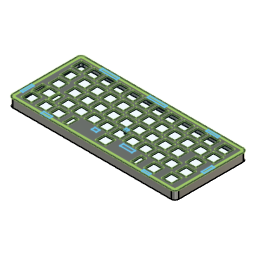
RowLow52V2-topcase v4 (Autodesk Fusion 360 design; units mm, degrees)
Autodesk Fusion 360 part; units mm, degrees
sketch "スケッチ1" plane through (0, 0, 0) normal (0, 0, 1) x (1, 0, 0)
  spline S0 degree 3 poles (2.4631, -100.8553) (0.8767, -100.8553) (-0.441, -99.5645) (-0.4745, -97.9777) knots 0 0 0 0 1 1 1 1
  line L0 (-0.4745, -97.9777) -> (-0.4745, -2.5093)
  spline S1 degree 3 poles (-0.4745, -2.5093) (-0.5048, -0.9017) (0.7856, 0.4413) (2.4031, 0.4748) knots 0 0 0 0 1 1 1 1
  line L1 (2.4031, 0.4748) -> (236.6144, 0.4695)
  spline S2 degree 3 poles (236.6144, 0.4695) (238.2009, 0.4695) (239.5181, -0.8213) (239.5513, -2.4081) knots 0 0 0 0 1 1 1 1
  line L2 (239.5513, -2.4081) -> (239.5337, -97.857)
  spline S3 degree 3 poles (239.5337, -97.857) (239.5643, -99.4643) (238.2739, -100.807) (236.6571, -100.8412) knots 0 0 0 0 1 1 1 1
  line L3 (236.6571, -100.8412) -> (2.4631, -100.8553)
  spline S4 degree 3 poles (2.4631, -103.3551) (-0.4734, -103.3554) (-2.9122, -100.9664) (-2.9739, -98.0302) knots 0 0 0 0 1 1 1 1
  line L4 (-2.9739, -98.0302) -> (-2.9746, -2.534)
  spline S5 degree 3 poles (-2.9746, -2.534) (-3.0134, 0.4445) (-0.6311, 2.9125) (2.3509, 2.9743) knots 0 0 0 0 1 1 1 1
  line L5 (2.3509, 2.9743) -> (236.614, 2.9697)
  spline S6 degree 3 poles (236.614, 2.9697) (239.5506, 2.9697) (241.9893, 0.5807) (242.0503, -2.3562) knots 0 0 0 0 1 1 1 1
  line L6 (242.0503, -2.3562) -> (242.0334, -97.8351)
  spline S7 degree 3 poles (242.0334, -97.8351) (242.0712, -100.8119) (239.6896, -103.2781) (236.7089, -103.3406) knots 0 0 0 0 1 1 1 1
  line L7 (236.7089, -103.3406) -> (2.4631, -103.3551)
  line L8 (239.0514, -2.4183) -> (239.0338, -97.857)
  spline S8 degree 3 poles (239.0338, -97.857) (239.0592, -99.2018) (237.9909, -100.3131) (236.6461, -100.3413) knots 0 0 0 0 1 1 1 1
  line L9 (236.6461, -100.3413) -> (2.51, -100.3547)
  spline S9 degree 3 poles (2.51, -100.3547) (1.1649, -100.3801) (0.0536, -99.3119) (0.0254, -97.9671) knots 0 0 0 0 1 1 1 1
  line L10 (0.0254, -97.9671) -> (0.0254, -2.5093)
  spline S10 degree 3 poles (0.0254, -2.5093) (0, -1.1645) (1.0682, -0.0529) (2.4134, -0.025) knots 0 0 0 0 1 1 1 1
  line L11 (2.4134, -0.025) -> (236.5671, -0.031)
  spline S11 degree 3 poles (236.5671, -0.031) (237.9119, -0.0053) (239.0235, -1.0739) (239.0514, -2.4183) knots 0 0 0 0 1 1 1 1
  line L12 (131.3131, -95.1177) -> (117.2132, -95.1177)
  line L13 (117.2132, -95.1177) -> (117.2132, -81.0175)
  line L14 (117.2132, -81.0175) -> (131.3131, -81.0175)
  line L15 (131.3131, -81.0175) -> (131.3131, -95.1177)
  line L16 (177.7735, -96.8678) -> (170.7734, -96.8678)
  line L17 (170.7734, -96.8678) -> (170.7734, -82.0678)
  line L18 (170.7734, -82.0678) -> (177.7735, -82.0678)
  line L19 (177.7735, -82.0678) -> (177.7735, -96.8678)
  line L20 (70.7531, -96.8678) -> (77.7533, -96.8678)
  line L21 (77.7533, -96.8678) -> (77.7533, -82.0678)
  line L22 (77.7533, -82.0678) -> (70.7531, -82.0678)
  line L23 (70.7531, -82.0678) -> (70.7531, -96.8678)
  line L24 (28.9193, -76.0677) -> (14.8195, -76.0677)
  line L25 (14.8195, -76.0677) -> (14.8195, -61.9675)
  line L26 (14.8195, -61.9675) -> (28.9197, -61.9675)
  line L27 (28.9197, -61.9675) -> (28.9193, -76.0677)
  line L28 (37.2696, -77.8178) -> (30.2694, -77.8178)
  line L29 (30.2694, -77.8178) -> (30.2694, -63.0178)
  line L30 (30.2694, -63.0178) -> (37.2696, -63.0178)
  line L31 (37.2696, -63.0178) -> (37.2696, -77.8178)
  line L32 (6.4696, -77.8178) -> (13.4698, -77.8178)
  line L33 (13.4698, -77.8178) -> (13.4698, -63.0178)
  line L34 (13.4698, -63.0178) -> (6.4696, -63.0178)
  line L35 (6.4696, -63.0178) -> (6.4696, -77.8178)
  line L36 (226.5634, -57.0177) -> (212.4632, -57.0177)
  line L37 (212.4632, -57.0177) -> (212.4632, -42.9175)
  line L38 (212.4632, -42.9175) -> (226.5634, -42.9175)
  line L39 (226.5634, -42.9175) -> (226.5634, -57.0177)
  line L40 (228.9443, -95.1177) -> (214.8445, -95.1177)
  line L41 (214.8445, -95.1177) -> (214.8445, -81.0175)
  line L42 (214.8445, -81.0175) -> (228.9443, -81.0175)
  line L43 (228.9443, -81.0175) -> (228.9443, -95.1177)
  line L44 (24.1568, -57.0177) -> (10.057, -57.0177)
  line L45 (10.057, -57.0177) -> (10.057, -42.9175)
  line L46 (10.057, -42.9175) -> (24.1572, -42.9175)
  line L47 (24.1572, -42.9175) -> (24.1568, -57.0177)
  line L48 (21.7756, -37.9677) -> (7.6761, -37.9677)
  line L49 (7.6761, -37.9677) -> (7.6761, -23.8675)
  line L50 (7.6761, -23.8675) -> (21.7759, -23.8675)
  line L51 (21.7759, -23.8675) -> (21.7756, -37.9677)
  line L52 (21.7756, -95.1177) -> (7.6761, -95.1177)
  line L53 (7.6761, -95.1177) -> (7.6761, -81.0175)
  line L54 (7.6761, -81.0175) -> (21.7759, -81.0175)
  line L55 (21.7759, -81.0175) -> (21.7756, -95.1177)
  line L56 (231.3259, -18.9177) -> (217.2257, -18.9177)
  line L57 (217.2257, -18.9177) -> (217.2257, -4.8175)
  line L58 (217.2257, -4.8175) -> (231.3259, -4.8175)
  line L59 (231.3259, -4.8175) -> (231.3259, -18.9177)
  line L60 (202.7509, -95.1177) -> (188.6507, -95.1177)
  line L61 (188.6507, -95.1177) -> (188.6507, -81.0175)
  line L62 (188.6507, -81.0175) -> (202.7509, -81.0175)
  line L63 (202.7509, -81.0175) -> (202.7509, -95.1177)
  line L64 (231.3259, -76.0677) -> (217.2257, -76.0677)
  line L65 (217.2257, -76.0677) -> (217.2257, -61.9675)
  line L66 (217.2257, -61.9675) -> (231.3259, -61.9675)
  line L67 (231.3259, -61.9675) -> (231.3259, -76.0677)
  line L68 (214.6568, -37.9677) -> (200.557, -37.9677)
  line L69 (200.557, -37.9677) -> (200.557, -23.8675)
  line L70 (200.557, -23.8675) -> (214.6568, -23.8675)
  line L71 (214.6568, -23.8675) -> (214.6568, -37.9677)
  line L72 (57.4943, -18.9177) -> (43.3941, -18.9177)
  line L73 (43.3941, -18.9177) -> (43.3941, -4.8175)
  line L74 (43.3941, -4.8175) -> (57.4943, -4.8175)
  line L75 (57.4943, -4.8175) -> (57.4943, -18.9177)
  line L76 (152.7443, -18.9177) -> (138.6441, -18.9177)
  line L77 (138.6441, -18.9177) -> (138.6441, -4.8175)
  line L78 (138.6441, -4.8175) -> (152.7443, -4.8175)
  line L79 (152.7443, -4.8175) -> (152.7443, -18.9177)
  line L80 (95.5943, -76.0677) -> (81.4941, -76.0677)
  line L81 (81.4941, -76.0677) -> (81.4941, -61.9675)
  line L82 (81.4941, -61.9675) -> (95.5943, -61.9675)
  line L83 (95.5943, -61.9675) -> (95.5943, -76.0677)
  line L84 (162.2693, -57.0177) -> (148.1691, -57.0177)
  line L85 (148.1691, -57.0177) -> (148.1691, -42.9175)
  line L86 (148.1691, -42.9175) -> (162.2693, -42.9175)
  line L87 (162.2693, -42.9175) -> (162.2693, -57.0177)
  line L88 (114.6443, -18.9177) -> (100.5441, -18.9177)
  line L89 (100.5441, -18.9177) -> (100.5441, -4.8175)
  line L90 (100.5441, -4.8175) -> (114.6443, -4.8175)
  line L91 (114.6443, -4.8175) -> (114.6443, -18.9177)
  line L92 (138.4568, -37.9677) -> (124.3566, -37.9677)
  line L93 (124.3566, -37.9677) -> (124.3566, -23.8675)
  line L94 (124.3566, -23.8675) -> (138.4568, -23.8675)
  line L95 (138.4568, -23.8675) -> (138.4568, -37.9677)
  line L96 (171.7943, -76.0677) -> (157.6945, -76.0677)
  line L97 (157.6945, -76.0677) -> (157.6945, -61.9675)
  line L98 (157.6945, -61.9675) -> (171.7943, -61.9675)
  line L99 (171.7943, -61.9675) -> (171.7943, -76.0677)
  line L100 (124.1693, -57.0177) -> (110.0691, -57.0177)
  line L101 (110.0691, -57.0177) -> (110.0691, -42.9175)
  line L102 (110.0691, -42.9175) -> (124.1693, -42.9175)
  line L103 (124.1693, -42.9175) -> (124.1693, -57.0177)
  line L104 (86.0693, -57.0177) -> (71.9691, -57.0177)
  line L105 (71.9691, -57.0177) -> (71.9691, -42.9175)
  line L106 (71.9691, -42.9175) -> (86.0693, -42.9175)
  line L107 (86.0693, -42.9175) -> (86.0693, -57.0177)
  line L108 (152.7443, -76.0677) -> (138.6441, -76.0677)
  line L109 (138.6441, -76.0677) -> (138.6441, -61.9675)
  line L110 (138.6441, -61.9675) -> (152.7443, -61.9675)
  line L111 (152.7443, -61.9675) -> (152.7443, -76.0677)
  line L112 (81.3068, -37.9677) -> (67.2066, -37.9677)
  line L113 (67.2066, -37.9677) -> (67.2066, -23.8675)
  line L114 (67.2066, -23.8675) -> (81.3068, -23.8675)
  line L115 (81.3068, -23.8675) -> (81.3068, -37.9677)
  line L116 (62.2568, -37.9677) -> (48.1566, -37.9677)
  line L117 (48.1566, -37.9677) -> (48.1566, -23.8675)
  line L118 (48.1566, -23.8675) -> (62.2568, -23.8675)
  line L119 (62.2568, -23.8675) -> (62.2568, -37.9677)
  line L120 (133.6943, -76.0677) -> (119.5941, -76.0677)
  line L121 (119.5941, -76.0677) -> (119.5941, -61.9675)
  line L122 (119.5941, -61.9675) -> (133.6943, -61.9675)
  line L123 (133.6943, -61.9675) -> (133.6943, -76.0677)
  line L124 (190.8443, -76.0677) -> (176.7445, -76.0677)
  line L125 (176.7445, -76.0677) -> (176.7445, -61.9675)
  line L126 (176.7445, -61.9675) -> (190.8443, -61.9675)
  line L127 (190.8443, -61.9675) -> (190.8443, -76.0677)
  line L128 (76.5443, -18.9177) -> (62.4441, -18.9177)
  line L129 (62.4441, -18.9177) -> (62.4441, -4.8175)
  line L130 (62.4441, -4.8175) -> (76.5443, -4.8175)
  line L131 (76.5443, -4.8175) -> (76.5443, -18.9177)
  line L132 (114.6443, -76.0677) -> (100.5441, -76.0677)
  line L133 (100.5441, -76.0677) -> (100.5441, -61.9675)
  line L134 (100.5441, -61.9675) -> (114.6443, -61.9675)
  line L135 (114.6443, -61.9675) -> (114.6443, -76.0677)
  line L136 (195.6068, -37.9677) -> (181.507, -37.9677)
  line L137 (181.507, -37.9677) -> (181.507, -23.8675)
  line L138 (181.507, -23.8675) -> (195.6068, -23.8675)
  line L139 (195.6068, -23.8675) -> (195.6068, -37.9677)
  line L140 (67.0193, -57.0177) -> (52.9191, -57.0177)
  line L141 (52.9191, -57.0177) -> (52.9191, -42.9175)
  line L142 (52.9191, -42.9175) -> (67.0193, -42.9175)
  line L143 (67.0193, -42.9175) -> (67.0193, -57.0177)
  line L144 (233.7068, -37.9677) -> (219.607, -37.9677)
  line L145 (219.607, -37.9677) -> (219.607, -23.8675)
  line L146 (219.607, -23.8675) -> (233.7068, -23.8675)
  line L147 (233.7068, -23.8675) -> (233.7068, -37.9677)
  line L148 (57.4943, -76.0677) -> (43.3941, -76.0677)
  line L149 (43.3941, -76.0677) -> (43.3941, -61.9675)
  line L150 (43.3941, -61.9675) -> (57.4943, -61.9675)
  line L151 (57.4943, -61.9675) -> (57.4943, -76.0677)
  line L152 (157.5068, -37.9677) -> (143.4066, -37.9677)
  line L153 (143.4066, -37.9677) -> (143.4066, -23.8675)
  line L154 (143.4066, -23.8675) -> (157.5068, -23.8675)
  line L155 (157.5068, -23.8675) -> (157.5068, -37.9677)
  line L156 (38.3007, -18.9138) -> (24.2006, -18.9138)
  line L157 (24.2006, -18.9138) -> (24.2006, -4.814)
  line L158 (24.2006, -4.814) -> (38.3007, -4.814)
  line L159 (38.3007, -4.814) -> (38.3007, -18.9138)
  line L160 (19.3943, -18.9177) -> (5.2945, -18.9177)
  line L161 (5.2945, -18.9177) -> (5.2945, -4.8175)
  line L162 (5.2945, -4.8175) -> (19.3947, -4.8175)
  line L163 (19.3947, -4.8175) -> (19.3943, -18.9177)
  line L164 (62.2568, -95.1177) -> (48.1566, -95.1177)
  line L165 (48.1566, -95.1177) -> (48.1566, -81.0175)
  line L166 (48.1566, -81.0175) -> (62.2568, -81.0175)
  line L167 (62.2568, -81.0175) -> (62.2568, -95.1177)
  line L168 (100.3568, -37.9677) -> (86.2566, -37.9677)
  line L169 (86.2566, -37.9677) -> (86.2566, -23.8675)
  line L170 (86.2566, -23.8675) -> (100.3568, -23.8675)
  line L171 (100.3568, -23.8675) -> (100.3568, -37.9677)
  line L172 (176.5568, -37.9677) -> (162.457, -37.9677)
  line L173 (162.457, -37.9677) -> (162.457, -23.8675)
  line L174 (162.457, -23.8675) -> (176.5568, -23.8675)
  line L175 (176.5568, -23.8675) -> (176.5568, -37.9677)
  line L176 (95.5943, -18.9177) -> (81.4941, -18.9177)
  line L177 (81.4941, -18.9177) -> (81.4941, -4.8175)
  line L178 (81.4941, -4.8175) -> (95.5943, -4.8175)
  line L179 (95.5943, -4.8175) -> (95.5943, -18.9177)
  line L180 (105.1193, -57.0177) -> (91.0191, -57.0177)
  line L181 (91.0191, -57.0177) -> (91.0191, -42.9175)
  line L182 (91.0191, -42.9175) -> (105.1193, -42.9175)
  line L183 (105.1193, -42.9175) -> (105.1193, -57.0177)
  line L184 (47.9693, -57.0177) -> (33.8695, -57.0177)
  line L185 (33.8695, -57.0177) -> (33.8695, -42.9175)
  line L186 (33.8695, -42.9175) -> (47.9697, -42.9175)
  line L187 (47.9697, -42.9175) -> (47.9693, -57.0177)
  line L188 (133.6943, -18.9177) -> (119.5941, -18.9177)
  line L189 (119.5941, -18.9177) -> (119.5941, -4.8175)
  line L190 (119.5941, -4.8175) -> (133.6943, -4.8175)
  line L191 (133.6943, -4.8175) -> (133.6943, -18.9177)
  line L192 (119.4068, -37.9677) -> (105.3066, -37.9677)
  line L193 (105.3066, -37.9677) -> (105.3066, -23.8675)
  line L194 (105.3066, -23.8675) -> (119.4068, -23.8675)
  line L195 (119.4068, -23.8675) -> (119.4068, -37.9677)
  line L196 (43.2068, -37.9677) -> (29.107, -37.9677)
  line L197 (29.107, -37.9677) -> (29.107, -23.8675)
  line L198 (29.107, -23.8675) -> (43.2072, -23.8675)
  line L199 (43.2072, -23.8675) -> (43.2068, -37.9677)
  line L200 (181.3193, -57.0177) -> (167.2195, -57.0177)
  line L201 (167.2195, -57.0177) -> (167.2195, -42.9175)
  line L202 (167.2195, -42.9175) -> (181.3193, -42.9175)
  line L203 (181.3193, -42.9175) -> (181.3193, -57.0177)
  line L204 (43.2068, -95.1177) -> (29.107, -95.1177)
  line L205 (29.107, -95.1177) -> (29.107, -81.0175)
  line L206 (29.107, -81.0175) -> (43.2072, -81.0175)
  line L207 (43.2072, -81.0175) -> (43.2068, -95.1177)
  line L208 (209.8943, -18.9177) -> (195.7945, -18.9177)
  line L209 (195.7945, -18.9177) -> (195.7945, -4.8175)
  line L210 (195.7945, -4.8175) -> (209.8943, -4.8175)
  line L211 (209.8943, -4.8175) -> (209.8943, -18.9177)
  line L212 (200.3693, -57.0177) -> (186.2695, -57.0177)
  line L213 (186.2695, -57.0177) -> (186.2695, -42.9175)
  line L214 (186.2695, -42.9175) -> (200.3693, -42.9175)
  line L215 (200.3693, -42.9175) -> (200.3693, -57.0177)
  line L216 (209.8943, -76.0677) -> (195.7945, -76.0677)
  line L217 (195.7945, -76.0677) -> (195.7945, -61.9675)
  line L218 (195.7945, -61.9675) -> (209.8943, -61.9675)
  line L219 (209.8943, -61.9675) -> (209.8943, -76.0677)
  line L220 (76.5443, -76.0677) -> (62.4441, -76.0677)
  line L221 (62.4441, -76.0677) -> (62.4441, -61.9675)
  line L222 (62.4441, -61.9675) -> (76.5443, -61.9675)
  line L223 (76.5443, -61.9675) -> (76.5443, -76.0677)
  line L224 (171.7943, -18.9177) -> (157.6945, -18.9177)
  line L225 (157.6945, -18.9177) -> (157.6945, -4.8175)
  line L226 (157.6945, -4.8175) -> (171.7943, -4.8175)
  line L227 (171.7943, -4.8175) -> (171.7943, -18.9177)
  line L228 (190.8443, -18.9177) -> (176.7445, -18.9177)
  line L229 (176.7445, -18.9177) -> (176.7445, -4.8175)
  line L230 (176.7445, -4.8175) -> (190.8443, -4.8175)
  line L231 (190.8443, -4.8175) -> (190.8443, -18.9177)
  line L232 (143.2193, -57.0177) -> (129.1191, -57.0177)
  line L233 (129.1191, -57.0177) -> (129.1191, -42.9175)
  line L234 (129.1191, -42.9175) -> (143.2193, -42.9175)
  line L235 (143.2193, -42.9175) -> (143.2193, -57.0177)
extrude "押し出し1" add sketch "スケッチ1" against normal blind 2 contours S0 L0 S1 L1 S2 L2 S3 L3 | L8 S8 L9 S9 L10 S10 L11 S11
extrude "押し出し2" add sketch "スケッチ1" against normal blind 12.1 contours S4 L4 S5 L5 S6 L6 S7 L7
sketch "スケッチ2" plane through (0, 0, 0) normal (0, 0, 1) x (1, 0, 0)
  line L0 (240, -43) -> (236, -43)
  line L1 (236, -43) -> (236, -58)
  line L2 (236, -58) -> (240, -58)
  line L3 (240, -58) -> (240, -43)
  line L4 (-1, -88) -> (2, -88)
  line L5 (2, -88) -> (2, -72)
  line L6 (2, -72) -> (-1, -72)
  line L7 (-1, -72) -> (-1, -88)
  line L8 (203.8666, 0.6445) -> (187.3492, 0.6445)
  line L9 (187.3492, 0.6445) -> (187.3492, -2.4525)
  line L10 (187.3492, -2.4525) -> (203.8666, -2.4525)
  line L11 (203.8666, -2.4525) -> (203.8666, 0.6445)
  line L12 (126, 1) -> (101, 1)
  line L13 (101, 1) -> (101, -3)
  line L14 (101, -3) -> (126, -3)
  line L15 (126, -3) -> (126, 1)
  line L16 (31, 1) -> (55, 1)
  line L17 (55, 1) -> (55, -3)
  line L18 (55, -3) -> (31, -3)
  line L19 (31, -3) -> (31, 1)
  line L20 (55, -97.4894) -> (42.5734, -97.4894)
  line L21 (42.5734, -97.4894) -> (42.5734, -101.8636)
  line L22 (42.5734, -101.8636) -> (55, -101.8636)
  line L23 (55, -101.8636) -> (55, -97.4894)
  line L24 (191, -101) -> (201, -101)
  line L25 (201, -101) -> (201, -98)
  line L26 (201, -98) -> (191, -98)
  line L27 (191, -98) -> (191, -101)
  line L28 (125, -58) -> (128.8943, -58)
  line L29 (128.8943, -58) -> (128.8943, -61.3754)
  line L30 (128.8943, -61.3754) -> (125, -61.3754)
  line L31 (125, -61.3754) -> (125, -58)
  constraint horizontal L0
  constraint vertical L1
  constraint horizontal L2
  constraint vertical L3
  constraint horizontal L4
  constraint vertical L5
  constraint horizontal L6
  constraint vertical L7
  constraint horizontal L8
  constraint vertical L9
  constraint horizontal L10
  constraint vertical L11
  constraint horizontal L12
  constraint vertical L13
  constraint horizontal L14
  constraint vertical L15
  constraint horizontal L16
  constraint vertical L17
  constraint horizontal L18
  constraint vertical L19
  constraint horizontal L20
  constraint vertical L21
  constraint horizontal L22
  constraint vertical L23
  constraint horizontal L24
  constraint vertical L25
  constraint horizontal L26
  constraint vertical L27
  constraint horizontal L28
  constraint vertical L29
  constraint horizontal L30
  constraint vertical L31
extrude "押し出し3" add sketch "スケッチ2" against normal blind 5
sketch "スケッチ3" plane through (-2.9746, 0, 0) normal (-1, -0.000007, 0) x (0.000007, -1, 0)
  line L0 (98.0302, 0) -> (2.534, 0)
  line L1 (2.534, 0) -> (2.534, -12.1)
  line L2 (2.534, -12.1) -> (98.0302, -12.1)
  line L3 (98.0302, -12.1) -> (98.0302, 0)
  line L4 (-3, 1) -> (26.2, 1)
  line L5 (26.2, -9.6) -> (35.597, -9.6)
  line L6 (35.6, -9.9177) -> (36.1, -9.9177)
  line L7 (26.2, -9.8487) -> (26.1782, -9.8487)
  line L8 (26.1782, -9.8487) -> (25.6889, -9.8487)
  line L9 (25.7, -8.6022) -> (36.1, -8.6022)
  line L10 (36.1, -8.6022) -> (36.1, -12.4)
  line L11 (36.1, -12.4) -> (25.7, -12.4)
  line L12 (25.7, -12.4) -> (25.7, -8.6022)
  dimension "d7" = 29.2
  dimension "d8" = 9.397
  constraint horizontal L4
  constraint horizontal L5
  constraint horizontal L6
  constraint horizontal L7
  constraint parallel L7 L8
  constraint horizontal L9
  constraint vertical L10
  constraint horizontal L11
  constraint vertical L12
  measures "d7" distance of L4.start L4.end
  measures "d8" distance of L5.start L5.end
sketch "スケッチ4" plane through (0, 0, 0) normal (1, 0, 0) x (0, 1, 0)
  line L0 (-29.5, 0) -> (-29.5, -8.6)
  constraint vertical L0
extrude "押し出し4" cut sketch "スケッチ3" against normal blind 6 contours L2 L9 L10 L12
sketch "スケッチ6" plane through (0, 0, 0) normal (0, 0, 1) x (1, 0, 0)
  line L0 (100.6144, -80) -> (107.4975, -80)
  line L1 (107.4975, -80) -> (107.4975, -85)
  line L2 (107.4975, -85) -> (100.6144, -85)
  line L3 (100.6144, -85) -> (100.6144, -80)
  line L4 (142.5654, -80) -> (160, -80)
  line L5 (160, -80) -> (160, -85)
  line L6 (160, -85) -> (142.5654, -85)
  line L7 (142.5654, -85) -> (142.5654, -80)
  constraint horizontal L0
  constraint vertical L1
  constraint horizontal L2
  constraint vertical L3
  constraint horizontal L4
  constraint vertical L5
  constraint horizontal L6
  constraint vertical L7
extrude "押し出し5" add sketch "スケッチ6" against normal blind 5 contours L4 L5 L6 L7
extrude "押し出し6" add sketch "スケッチ6" against normal blind 5 contours L0 L1 L2 L3
sketch "スケッチ5" plane through (0, 0, 0) normal (0, 0, 1) x (1, 0, 0)
  line L0 (42.1306, -60.1098) -> (228.9193, -60.1098)
  line L1 (228.9193, -60.1098) -> (228.9193, -59.0023)
  line L2 (228.9193, -59.0023) -> (42.1306, -59.0023)
  line L3 (42.1306, -59.0023) -> (42.1306, -60.1098)
  line L4 (212.8136, -23.1698) -> (212.8136, -20.6148)
  line L5 (38.8528, -20.6148) -> (38.8528, -23.1698)
  constraint horizontal L0
  constraint vertical L1
  constraint horizontal L2
  constraint vertical L3
  constraint vertical L5
